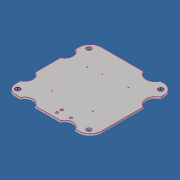
# Autodesk Inventor part: Eagle PCB rev 21
Saved by Autodesk Inventor 2016 (Build 200138000, 138)
## iProperties
Created: 2015-07-16
Part Number: Eagle PCB rev 21
Material: Generic
Document SubType Name: Modeling
Designer: Samuel Clay
Density: 1 g/cm^3
Appearance: Default
Author: Samuel Clay
Autodesk Inventor part; units mm, degrees
ref_plane "YZ Plane" through (0, 0, 0) normal (1, 0, 0) x (0, 1, 0)
ref_plane "XZ Plane" through (0, 0, 0) normal (0, 1, 0) x (-1, 0, 0)
ref_plane "XY Plane" through (0, 0, 0) normal (0, 0, 1) x (1, 0, 0)
sketch "Sketch1" plane through (0, 0, 0) normal (0, 0, 1) x (1, 0, 0)
  point P0 (0, 0)
sketch "0" plane through (0, 0, 0) normal (0, 1, 0) x (-1, 0, 0)
  line L0 (13.7795, -8.8674) -> (14.0221, -8.6401)
  line L1 (-19.1035, -9.4795) -> (-18.8376, -9.6291)
  line L2 (-20.445, -8.2504) -> (-20.2566, -8.4904)
  line L3 (3.0378, 26.1029) -> (3.2455, 25.8302)
  line L4 (3.2455, 25.8302) -> (3.4787, 25.5788)
  line L5 (-20.6394, 24.162) -> (-20.7961, 23.8688)
  line L6 (14.6382, 14.4375) -> (14.9109, 14.2297)
  line L7 (13.5247, 16.1335) -> (13.6387, 15.8102)
  line L8 (13.4425, 17.8296) -> (13.3929, 17.4904)
  line L9 (-21.0504, 23.2549) -> (-21.1469, 22.9368)
  line L10 (-19.8321, 25.2141) -> (-20.0593, 24.9715)
  line L11 (-19.5894, 25.4413) -> (-19.8321, 25.2141)
  line L12 (14.3869, 14.6706) -> (14.6382, 14.4375)
  line L13 (-16.5722, 26.6911) -> (-16.903, 26.6585)
  line L14 (-17.1381, 24.416) -> (-17.51, 24.7879)
  line L15 (-17.51, 24.7879) -> (-18.018, 24.924)
  line L16 (-18.8979, 23.4) -> (-18.526, 23.0281)
  line L17 (-18.018, 24.924) -> (-18.526, 24.7879)
  line L18 (-18.526, 24.7879) -> (-18.8979, 24.416)
  line L19 (-18.8979, 24.416) -> (-19.034, 23.908)
  line L20 (-19.034, 23.908) -> (-18.8979, 23.4)
  line L21 (-18.526, 23.0281) -> (-18.018, 22.892)
  line L22 (-18.018, 22.892) -> (-17.51, 23.0281)
  line L23 (14.3869, 19.6254) -> (14.1592, 19.369)
  line L24 (-19.0623, 25.8458) -> (-19.3325, 25.6522)
  line L25 (13.5247, 18.1624) -> (13.4425, 17.8296)
  line L26 (-20.2702, 24.7145) -> (-20.4638, 24.4443)
  line L27 (13.4425, 16.4663) -> (13.5247, 16.1335)
  line L28 (13.7834, 15.4994) -> (13.9574, 15.2041)
  line L29 (-19.3591, -9.3127) -> (-19.1035, -9.4795)
  line L30 (15.4666, -5.7111) -> (15.4992, -5.3803)
  line L31 (-4.9959, 24.162) -> (-4.81, 23.976)
  line L32 (-4.556, 24.924) -> (-4.81, 24.8559)
  line L33 (-4.81, 24.8559) -> (-4.9959, 24.67)
  line L34 (-4.9959, 24.67) -> (-5.064, 24.416)
  line L35 (-5.064, 24.416) -> (-4.9959, 24.162)
  line L36 (-4.81, 23.976) -> (-4.556, 23.908)
  line L37 (-4.556, 23.908) -> (-4.302, 23.976)
  line L38 (-4.302, 23.976) -> (-4.116, 24.162)
  line L39 (-4.116, 24.162) -> (-4.048, 24.416)
  line L40 (-10.487, -0.73) -> (-10.5091, -0.6475)
  line L41 (-10.5091, -0.8125) -> (-10.487, -0.73)
  line L42 (-10.5695, -0.8729) -> (-10.5091, -0.8125)
  line L43 (-10.652, -0.895) -> (-10.5695, -0.8729)
  line L44 (-10.7345, -0.8729) -> (-10.652, -0.895)
  line L45 (-10.7949, -0.8125) -> (-10.7345, -0.8729)
  line L46 (-10.817, -0.73) -> (-10.7949, -0.8125)
  line L47 (-10.7949, -0.6475) -> (-10.817, -0.73)
  line L48 (-10.7345, -0.5871) -> (-10.7949, -0.6475)
  line L49 (-10.652, -0.565) -> (-10.7345, -0.5871)
  line L50 (-10.5695, -0.5871) -> (-10.652, -0.565)
  line L51 (-10.5091, -0.6475) -> (-10.5695, -0.5871)
  line L52 (-18.2793, -9.8747) -> (-17.9893, -9.9696)
  line L53 (4.842, 17.469) -> (4.7595, 17.4469)
  line L54 (4.7595, 17.4469) -> (4.6991, 17.3865)
  line L55 (4.6991, 17.3865) -> (4.677, 17.304)
  line L56 (4.677, 17.304) -> (4.6991, 17.2215)
  line L57 (4.7595, 17.1611) -> (4.842, 17.139)
  line L58 (4.842, 17.139) -> (4.9245, 17.1611)
  line L59 (4.9245, 17.1611) -> (4.9849, 17.2215)
  line L60 (4.9849, 17.2215) -> (5.007, 17.304)
  line L61 (-21.32, -4.136) -> (-21.32, -6.0009)
  line L62 (-9.89, 22.96) -> (-9.636, 22.892)
  line L63 (-9.636, 22.892) -> (-9.382, 22.96)
  line L64 (-9.382, 22.96) -> (-9.196, 23.146)
  line L65 (-9.196, 23.146) -> (-9.128, 23.4)
  line L66 (-9.128, 23.4) -> (-9.196, 23.654)
  line L67 (-10.0759, 23.146) -> (-9.89, 22.96)
  line L68 (-10.144, 23.4) -> (-10.0759, 23.146)
  line L69 (-10.0759, 23.654) -> (-10.144, 23.4)
  line L70 (-9.89, 23.8399) -> (-10.0759, 23.654)
  line L71 (-9.636, 23.908) -> (-9.89, 23.8399)
  line L72 (-9.382, 23.8399) -> (-9.636, 23.908)
  line L73 (-9.196, 23.654) -> (-9.382, 23.8399)
  line L74 (4.3075, 24.9753) -> (4.6183, 24.8306)
  line L75 (14.4603, -8.1405) -> (14.6539, -7.8703)
  line L76 (14.6539, -7.8703) -> (14.8294, -7.588)
  line L77 (-17.9893, -9.9696) -> (-17.6937, -10.0453)
  line L78 (-8.8595, 25.8302) -> (-8.6517, 26.1029)
  line L79 (-8.6517, 26.1029) -> (-8.4713, 26.3944)
  line L80 (12.0629, -9.8584) -> (12.3741, -9.7413)
  line L81 (-18.5625, -9.761) -> (-18.2793, -9.8747)
  line L82 (-19.542, -7.08) -> (-19.4059, -7.588)
  line L83 (15.51, -5.048) -> (15.51, -3.628)
  line L84 (14.8294, -7.588) -> (14.9861, -7.2949)
  line L85 (14.9861, -7.2949) -> (15.1233, -6.9921)
  line L86 (15.1233, -6.9921) -> (15.2404, -6.6809)
  line L87 (14.0221, -8.6401) -> (14.2494, -8.3975)
  line L88 (-19.4059, -7.588) -> (-19.034, -7.9599)
  line L89 (-18.526, -6.064) -> (-19.034, -6.2002)
  line L90 (-19.034, -6.2002) -> (-19.4059, -6.572)
  line L91 (-17.0909, -10.1381) -> (-16.7862, -10.1547)
  line L92 (-4.302, 24.8559) -> (-4.556, 24.924)
  line L93 (-8.4713, 26.3944) -> (-8.32, 26.702)
  line L94 (-17.51, -7.08) -> (-17.6461, -6.572)
  line L95 (-14.4882, 26.1029) -> (-14.2805, 25.8302)
  line L96 (-12.5844, 24.7167) -> (-12.2516, 24.6345)
  line L97 (-14.6686, 26.3944) -> (-14.4882, 26.1029)
  line L98 (-19.4059, -6.572) -> (-19.542, -7.08)
  line L99 (7.2938, 24.8306) -> (7.6046, 24.9753)
  line L100 (4.9245, 17.4469) -> (4.842, 17.469)
  line L101 (4.6991, 17.2215) -> (4.7595, 17.1611)
  line L102 (14.2494, -8.3975) -> (14.4603, -8.1405)
  line L103 (-13.5139, 25.1494) -> (-13.2185, 24.9753)
  line L104 (-13.2185, 24.9753) -> (-12.9077, 24.8306)
  line L105 (2.706, 26.702) -> (2.8574, 26.3944)
  line L106 (15.3369, -6.3628) -> (15.4124, -6.0391)
  line L107 (15.4124, -6.0391) -> (15.4666, -5.7111)
  line L108 (-16.7862, -10.1547) -> (-16.4811, -10.1513)
  line L109 (-9.9214, 24.9753) -> (-9.6261, 25.1494)
  line L110 (-13.791, 25.3512) -> (-13.5139, 25.1494)
  line L111 (-14.82, 26.702) -> (-14.6686, 26.3944)
  line L112 (-17.6937, -10.0453) -> (-17.3938, -10.1016)
  line L113 (6.6377, 24.6345) -> (6.9705, 24.7167)
  line L114 (6.9705, 24.7167) -> (7.2938, 24.8306)
  line L115 (-20.0529, -8.7176) -> (-19.8348, -8.931)
  line L116 (-11.8395, 16.1769) -> (-11.922, 16.199)
  line L117 (-12.0649, 15.9515) -> (-12.0045, 15.8911)
  line L118 (-11.922, 16.199) -> (-12.0045, 16.1769)
  line L119 (-11.9124, 24.5849) -> (-11.57, 24.5683)
  line L120 (-11.57, 24.5683) -> (-11.2276, 24.5849)
  line L121 (4.6183, 24.8306) -> (4.9416, 24.7167)
  line L122 (7.6046, 24.9753) -> (7.8999, 25.1494)
  line L123 (4.9416, 24.7167) -> (5.2744, 24.6345)
  line L124 (-20.6173, -7.9986) -> (-20.445, -8.2504)
  line L125 (-21.32, 21.622) -> (-21.32, 3.38)
  line L126 (-12.0045, 16.1769) -> (-12.0649, 16.1165)
  line L127 (-12.0649, 16.1165) -> (-12.087, 16.034)
  line L128 (-11.757, 16.034) -> (-11.7791, 16.1165)
  line L129 (-11.7791, 15.9515) -> (-11.757, 16.034)
  line L130 (-11.8395, 15.8911) -> (-11.7791, 15.9515)
  line L131 (-11.922, 15.869) -> (-11.8395, 15.8911)
  line L132 (-12.0045, 15.8911) -> (-11.922, 15.869)
  line L133 (-12.087, 16.034) -> (-12.0649, 15.9515)
  line L134 (-11.7791, 16.1165) -> (-11.8395, 16.1769)
  line L135 (4.9849, 17.3865) -> (4.9245, 17.4469)
  line L136 (5.007, 17.304) -> (4.9849, 17.3865)
  line L137 (-16.1769, -10.128) -> (-15.328, -10.128)
  line L138 (3.735, 25.3512) -> (4.0121, 25.1494)
  line L139 (4.0121, 25.1494) -> (4.3075, 24.9753)
  line L140 (5.6136, 24.5849) -> (5.956, 24.5683)
  line L141 (5.956, 24.5683) -> (6.2984, 24.5849)
  line L142 (2.8574, 26.3944) -> (3.0378, 26.1029)
  line L143 (-17.6461, -7.588) -> (-17.51, -7.08)
  line L144 (-18.018, -7.9599) -> (-17.6461, -7.588)
  line L145 (-18.526, -8.096) -> (-18.018, -7.9599)
  line L146 (-19.034, -7.9599) -> (-18.526, -8.096)
  line L147 (-18.018, -6.2002) -> (-18.526, -6.064)
  line L148 (-17.6461, -6.572) -> (-18.018, -6.2002)
  line L149 (13.5225, -9.0783) -> (13.7795, -8.8674)
  line L150 (-20.7727, -7.736) -> (-20.6173, -7.9986)
  line L151 (-4.048, 22.384) -> (-4.116, 22.638)
  line L152 (6.277, 0.54) -> (6.2549, 0.6225)
  line L153 (6.2549, 0.4575) -> (6.277, 0.54)
  line L154 (6.1945, 0.3971) -> (6.2549, 0.4575)
  line L155 (6.112, 0.375) -> (6.1945, 0.3971)
  line L156 (6.0295, 0.3971) -> (6.112, 0.375)
  line L157 (5.9691, 0.4575) -> (6.0295, 0.3971)
  line L158 (5.947, 0.54) -> (5.9691, 0.4575)
  line L159 (5.9691, 0.6225) -> (5.947, 0.54)
  line L160 (6.0295, 0.6829) -> (5.9691, 0.6225)
  line L161 (6.112, 0.705) -> (6.0295, 0.6829)
  line L162 (6.1945, 0.6829) -> (6.112, 0.705)
  line L163 (6.2549, 0.6225) -> (6.1945, 0.6829)
  line L164 (8.4334, 25.5788) -> (8.6665, 25.8302)
  line L165 (8.6665, 25.8302) -> (8.8743, 26.1029)
  line L166 (-4.116, 22.638) -> (-4.302, 22.8239)
  line L167 (-20.2566, -8.4904) -> (-20.0529, -8.7176)
  line L168 (-4.302, 22.8239) -> (-4.556, 22.892)
  line L169 (-4.9959, 22.13) -> (-4.81, 21.944)
  line L170 (-4.556, 22.892) -> (-4.81, 22.8239)
  line L171 (-4.81, 22.8239) -> (-4.9959, 22.638)
  line L172 (-4.9959, 22.638) -> (-5.064, 22.384)
  line L173 (-5.064, 22.384) -> (-4.9959, 22.13)
  line L174 (-4.81, 21.944) -> (-4.556, 21.876)
  line L175 (-4.556, 21.876) -> (-4.302, 21.944)
  line L176 (-4.302, 21.944) -> (-4.116, 22.13)
  line L177 (-4.116, 22.13) -> (-4.048, 22.384)
  line L178 (13.2435, 26.2829) -> (13.0013, 26.3926)
  line L179 (13.0013, 26.3926) -> (12.7524, 26.4863)
  line L180 (-20.0212, -3.2426) -> (-19.758, -2.9462)
  line L181 (-19.758, -2.9462) -> (-19.5247, -2.6258)
  line L182 (-19.5247, -2.6258) -> (-19.3234, -2.2843)
  line L183 (-15.1529, -9.7724) -> (-15.328, -10.128)
  line L184 (15.2024, -3.4767) -> (15.51, -3.628)
  line L185 (-14.9443, -9.4353) -> (-15.1529, -9.7724)
  line L186 (13.6387, 0.9597) -> (13.5247, 0.6364)
  line L187 (-14.7041, -9.1199) -> (-14.9443, -9.4353)
  line L188 (14.9109, -3.2963) -> (15.2024, -3.4767)
  line L189 (-14.4346, -8.8293) -> (-14.7041, -9.1199)
  line L190 (13.7834, 1.2705) -> (13.6387, 0.9597)
  line L191 (-14.1382, -8.5661) -> (-14.4346, -8.8293)
  line L192 (-13.8177, -8.3328) -> (-14.1382, -8.5661)
  line L193 (14.6382, -3.0885) -> (14.9109, -3.2963)
  line L194 (-13.4762, -8.1315) -> (-13.8177, -8.3328)
  line L195 (14.3869, -2.8554) -> (14.6382, -3.0885)
  line L196 (-13.1168, -7.9642) -> (-13.4762, -8.1315)
  line L197 (-12.743, -7.8324) -> (-13.1168, -7.9642)
  line L198 (-12.3581, -7.7374) -> (-12.743, -7.8324)
  line L199 (-11.9659, -7.68) -> (-12.3581, -7.7374)
  line L200 (13.9574, 1.5659) -> (13.7834, 1.2705)
  line L201 (14.1592, -2.5991) -> (14.3869, -2.8554)
  line L202 (-11.57, -7.6608) -> (-11.9659, -7.68)
  line L203 (13.9574, -2.3219) -> (14.1592, -2.5991)
  line L204 (-11.174, -7.68) -> (-11.57, -7.6608)
  line L205 (14.1592, 1.843) -> (13.9574, 1.5659)
  line L206 (13.7834, -2.0266) -> (13.9574, -2.3219)
  line L207 (-10.7818, -7.7374) -> (-11.174, -7.68)
  line L208 (14.3869, 2.0993) -> (14.1592, 1.843)
  line L209 (-10.397, -7.8324) -> (-10.7818, -7.7374)
  line L210 (-10.0231, -7.9642) -> (-10.397, -7.8324)
  line L211 (-9.6637, -8.1315) -> (-10.0231, -7.9642)
  line L212 (-9.3222, -8.3328) -> (-9.6637, -8.1315)
  line L213 (14.6382, 2.3325) -> (14.3869, 2.0993)
  line L214 (13.6387, -1.7158) -> (13.7834, -2.0266)
  line L215 (-9.0018, -8.5661) -> (-9.3222, -8.3328)
  line L216 (-8.7054, -8.8293) -> (-9.0018, -8.5661)
  line L217 (13.5247, -1.3925) -> (13.6387, -1.7158)
  line L218 (14.9109, 2.5402) -> (14.6382, 2.3325)
  line L219 (-8.4358, -9.1199) -> (-8.7054, -8.8293)
  line L220 (13.4425, -1.0597) -> (13.5247, -1.3925)
  line L221 (-8.1956, -9.4353) -> (-8.4358, -9.1199)
  line L222 (15.2024, 2.7206) -> (14.9109, 2.5402)
  line L223 (-7.987, -9.7724) -> (-8.1956, -9.4353)
  line L224 (13.3929, -0.7205) -> (13.4425, -1.0597)
  line L225 (-7.812, -10.128) -> (-7.987, -9.7724)
  line L226 (-20.9643, 3.2049) -> (-21.32, 3.38)
  line L227 (13.3763, -0.378) -> (13.3929, -0.7205)
  line L228 (-20.6272, 2.9963) -> (-20.9643, 3.2049)
  line L229 (-20.3119, 2.7561) -> (-20.6272, 2.9963)
  line L230 (-20.0212, 2.4866) -> (-20.3119, 2.7561)
  line L231 (13.3929, -0.0356) -> (13.3763, -0.378)
  line L232 (-19.758, 2.1902) -> (-20.0212, 2.4866)
  line L233 (15.51, 2.872) -> (15.2024, 2.7206)
  line L234 (13.4425, 0.3036) -> (13.3929, -0.0356)
  line L235 (13.5247, 0.6364) -> (13.4425, 0.3036)
  line L236 (-19.5247, 1.8697) -> (-19.758, 2.1902)
  line L237 (-19.3234, 1.5282) -> (-19.5247, 1.8697)
  line L238 (-20.9333, 23.566) -> (-21.0504, 23.2549)
  line L239 (13.9574, 15.2041) -> (14.1592, 14.9269)
  line L240 (-17.002, 23.908) -> (-17.1381, 24.416)
  line L241 (-21.3091, 21.9542) -> (-21.32, 21.622)
  line L242 (-17.1381, 23.4) -> (-17.002, 23.908)
  line L243 (-17.51, 23.0281) -> (-17.1381, 23.4)
  line L244 (-20.4638, 24.4443) -> (-20.6394, 24.162)
  line L245 (14.6382, 19.8585) -> (14.3869, 19.6254)
  line L246 (15.51, 20.398) -> (15.2024, 20.2466)
  line L247 (-17.8729, 26.4324) -> (-18.184, 26.3153)
  line L248 (13.3929, 16.8056) -> (13.4425, 16.4663)
  line L249 (-20.7961, 23.8688) -> (-20.9333, 23.566)
  line L250 (-18.4868, 26.1781) -> (-18.78, 26.0214)
  line L251 (-18.78, 26.0214) -> (-19.0623, 25.8458)
  line L252 (-21.1469, 22.9368) -> (-21.2224, 22.613)
  line L253 (13.732, -6.826) -> (13.5959, -6.318)
  line L254 (13.3763, 17.148) -> (13.3929, 16.8056)
  line L255 (13.3929, 17.4904) -> (13.3763, 17.148)
  line L256 (-18.184, 26.3153) -> (-18.4868, 26.1781)
  line L257 (-19.3325, 25.6522) -> (-19.5894, 25.4413)
  line L258 (14.1592, 19.369) -> (13.9574, 19.0919)
  line L259 (13.6387, 15.8102) -> (13.7834, 15.4994)
  line L260 (-21.2765, 22.285) -> (-21.3091, 21.9542)
  line L261 (-21.2224, 22.613) -> (-21.2765, 22.285)
  line L262 (-17.5548, 26.5289) -> (-17.8729, 26.4324)
  line L263 (-20.0593, 24.9715) -> (-20.2702, 24.7145)
  line L264 (-17.231, 26.6044) -> (-17.5548, 26.5289)
  line L265 (15.2024, 20.2466) -> (14.9109, 20.0662)
  line L266 (14.9109, 20.0662) -> (14.6382, 19.8585)
  line L267 (-16.24, 26.702) -> (-16.5722, 26.6911)
  line L268 (-16.903, 26.6585) -> (-17.231, 26.6044)
  line L269 (14.9109, 14.2297) -> (15.2024, 14.0493)
  line L270 (15.2024, 14.0493) -> (15.51, 13.898)
  line L271 (13.5959, -6.318) -> (13.224, -5.9462)
  line L272 (13.224, -5.9462) -> (12.716, -5.81)
  line L273 (11.8362, -7.334) -> (12.208, -7.7059)
  line L274 (14.1592, 14.9269) -> (14.3869, 14.6706)
  line L275 (13.6387, 18.4857) -> (13.5247, 18.1624)
  line L276 (13.9574, 19.0919) -> (13.7834, 18.7965)
  line L277 (13.7834, 18.7965) -> (13.6387, 18.4857)
  line L278 (12.716, -5.81) -> (12.208, -5.9462)
  line L279 (12.208, -5.9462) -> (11.8362, -6.318)
  line L280 (11.8362, -6.318) -> (11.7, -6.826)
  line L281 (11.7, -6.826) -> (11.8362, -7.334)
  line L282 (12.208, -7.7059) -> (12.716, -7.842)
  line L283 (12.716, -7.842) -> (13.224, -7.7059)
  line L284 (13.224, -7.7059) -> (13.5959, -7.334)
  line L285 (13.5959, -7.334) -> (13.732, -6.826)
  line L286 (13.986, 24.162) -> (13.8499, 24.67)
  line L287 (13.8499, 24.67) -> (13.478, 25.0419)
  line L288 (13.478, 25.0419) -> (12.97, 25.178)
  line L289 (12.0902, 23.654) -> (12.462, 23.2821)
  line L290 (12.97, 25.178) -> (12.462, 25.0419)
  line L291 (12.462, 25.0419) -> (12.0902, 24.67)
  line L292 (12.0902, 24.67) -> (11.954, 24.162)
  line L293 (11.954, 24.162) -> (12.0902, 23.654)
  line L294 (12.462, 23.2821) -> (12.97, 23.146)
  line L295 (-14.82, 26.702) -> (-16.24, 26.702)
  line L296 (12.97, 23.146) -> (13.478, 23.2821)
  line L297 (13.478, 23.2821) -> (13.8499, 23.654)
  line L298 (13.8499, 23.654) -> (13.986, 24.162)
  line L299 (-14.2805, 25.8302) -> (-14.0473, 25.5788)
  line L300 (-14.0473, 25.5788) -> (-13.791, 25.3512)
  line L301 (-12.9077, 24.8306) -> (-12.5844, 24.7167)
  line L302 (-12.2516, 24.6345) -> (-11.9124, 24.5849)
  line L303 (-11.2276, 24.5849) -> (-10.8883, 24.6345)
  line L304 (-10.8883, 24.6345) -> (-10.5555, 24.7167)
  line L305 (-10.5555, 24.7167) -> (-10.2322, 24.8306)
  line L306 (-10.2322, 24.8306) -> (-9.9214, 24.9753)
  line L307 (-9.6261, 25.1494) -> (-9.3489, 25.3512)
  line L308 (-9.3489, 25.3512) -> (-9.0926, 25.5788)
  line L309 (-9.0926, 25.5788) -> (-8.8595, 25.8302)
  line L310 (2.706, 26.702) -> (-8.32, 26.702)
  line L311 (3.4787, 25.5788) -> (3.735, 25.3512)
  line L312 (5.2744, 24.6345) -> (5.6136, 24.5849)
  line L313 (6.2984, 24.5849) -> (6.6377, 24.6345)
  line L314 (7.8999, 25.1494) -> (8.1771, 25.3512)
  line L315 (8.1771, 25.3512) -> (8.4334, 25.5788)
  line L316 (8.8743, 26.1029) -> (9.0547, 26.3944)
  line L317 (9.0547, 26.3944) -> (9.206, 26.702)
  line L318 (11.446, 26.702) -> (9.206, 26.702)
  line L319 (11.7118, 26.6933) -> (11.446, 26.702)
  line L320 (11.9765, 26.6672) -> (11.7118, 26.6933)
  line L321 (12.2389, 26.6239) -> (11.9765, 26.6672)
  line L322 (12.4979, 26.5635) -> (12.2389, 26.6239)
  line L323 (12.7524, 26.4863) -> (12.4979, 26.5635)
  line L324 (13.478, 26.1575) -> (13.2435, 26.2829)
  line L325 (13.7039, 26.0171) -> (13.478, 26.1575)
  line L326 (13.92, 25.8622) -> (13.7039, 26.0171)
  line L327 (14.1256, 25.6935) -> (13.92, 25.8622)
  line L328 (14.3197, 25.5117) -> (14.1256, 25.6935)
  line L329 (14.5015, 25.3176) -> (14.3197, 25.5117)
  line L330 (14.6702, 25.112) -> (14.5015, 25.3176)
  line L331 (14.8251, 24.8958) -> (14.6702, 25.112)
  line L332 (14.9656, 24.67) -> (14.8251, 24.8958)
  line L333 (15.0909, 24.4354) -> (14.9656, 24.67)
  line L334 (15.2007, 24.1932) -> (15.0909, 24.4354)
  line L335 (15.2944, 23.9443) -> (15.2007, 24.1932)
  line L336 (15.3716, 23.6898) -> (15.2944, 23.9443)
  line L337 (15.4319, 23.4308) -> (15.3716, 23.6898)
  line L338 (15.4753, 23.1684) -> (15.4319, 23.4308)
  line L339 (15.5013, 22.9038) -> (15.4753, 23.1684)
  line L340 (15.51, 22.638) -> (15.5013, 22.9038)
  line L341 (15.51, 20.398) -> (15.51, 22.638)
  line L342 (15.51, 2.872) -> (15.51, 13.898)
  line L343 (15.4992, -5.3803) -> (15.51, -5.048)
  line L344 (15.2404, -6.6809) -> (15.3369, -6.3628)
  line L345 (13.2523, -9.2719) -> (13.5225, -9.0783)
  line L346 (12.97, -9.4474) -> (13.2523, -9.2719)
  line L347 (12.6769, -9.6041) -> (12.97, -9.4474)
  line L348 (12.3741, -9.7413) -> (12.6769, -9.6041)
  line L349 (11.7448, -9.9549) -> (12.0629, -9.8584)
  line L350 (11.4211, -10.0304) -> (11.7448, -9.9549)
  line L351 (11.0931, -10.0846) -> (11.4211, -10.0304)
  line L352 (10.7623, -10.1172) -> (11.0931, -10.0846)
  line L353 (10.43, -10.128) -> (10.7623, -10.1172)
  line L354 (-7.812, -10.128) -> (10.43, -10.128)
  line L355 (-16.4811, -10.1513) -> (-16.1769, -10.128)
  line L356 (-17.3938, -10.1016) -> (-17.0909, -10.1381)
  line L357 (-18.8376, -9.6291) -> (-18.5625, -9.761)
  line L358 (-19.6032, -9.1297) -> (-19.3591, -9.3127)
  line L359 (-19.8348, -8.931) -> (-19.6032, -9.1297)
  line L360 (-20.9107, -7.4639) -> (-20.7727, -7.736)
  line L361 (-21.0306, -7.1833) -> (-20.9107, -7.4639)
  line L362 (-21.1318, -6.8954) -> (-21.0306, -7.1833)
  line L363 (-21.214, -6.6016) -> (-21.1318, -6.8954)
  line L364 (-21.2768, -6.303) -> (-21.214, -6.6016)
  line L365 (-21.32, -6.0009) -> (-21.2768, -6.303)
  line L366 (-21.32, -4.136) -> (-20.9643, -3.961)
  line L367 (-20.9643, -3.961) -> (-20.6272, -3.7524)
  line L368 (-20.6272, -3.7524) -> (-20.3119, -3.5122)
  line L369 (-20.3119, -3.5122) -> (-20.0212, -3.2426)
  line L370 (-19.3234, -2.2843) -> (-19.1561, -1.9249)
  line L371 (-19.1561, -1.9249) -> (-19.0243, -1.551)
  line L372 (-19.0243, -1.551) -> (-18.9293, -1.1662)
  line L373 (-18.9293, -1.1662) -> (-18.872, -0.774)
  line L374 (-18.872, -0.774) -> (-18.8528, -0.378)
  line L375 (-18.8528, -0.378) -> (-18.872, 0.0179)
  line L376 (-18.872, 0.0179) -> (-18.9293, 0.4101)
  line L377 (-18.9293, 0.4101) -> (-19.0243, 0.795)
  line L378 (-19.0243, 0.795) -> (-19.1561, 1.1688)
  line L379 (-19.1561, 1.1688) -> (-19.3234, 1.5282)
  line L380 (-4.048, 24.416) -> (-4.116, 24.67)
  line L381 (-4.116, 24.67) -> (-4.302, 24.8559)
  dimension "d0" = 36.83
  constraints: 764 end point, 165 perpendicular, 137 parallel, 4 collinear
  measures "d0" distance between parallel lines of L342 L125
extrude "Extrusion1" add sketch "0" along normal blind 0.7112
sketch "Sketch3" plane through (0, 0.7112, 0) normal (0, 1, 0) x (1, 0, 0)
  line L0 (-13.986, -24.162) -> (-13.8499, -23.654) projected
  line L1 (-13.8499, -23.654) -> (-13.478, -23.2821) projected
  line L2 (-13.478, -23.2821) -> (-12.97, -23.146) projected
  line L3 (-12.97, -23.146) -> (-12.462, -23.2821) projected
  line L4 (-12.462, -23.2821) -> (-12.0902, -23.654) projected
  line L5 (-12.0902, -23.654) -> (-11.954, -24.162) projected
  line L6 (-11.954, -24.162) -> (-12.0902, -24.67) projected
  line L7 (-12.0902, -24.67) -> (-12.462, -25.0419) projected
  line L8 (-12.462, -25.0419) -> (-12.97, -25.178) projected
  line L9 (-12.97, -25.178) -> (-13.478, -25.0419) projected
  line L10 (-13.478, -25.0419) -> (-13.8499, -24.67) projected
  line L11 (-13.8499, -24.67) -> (-13.986, -24.162) projected
  line L12 (-13.732, 6.826) -> (-13.5959, 7.334) projected
  line L13 (-13.5959, 7.334) -> (-13.224, 7.7059) projected
  line L14 (-13.224, 7.7059) -> (-12.716, 7.842) projected
  line L15 (-12.716, 7.842) -> (-12.208, 7.7059) projected
  line L16 (-12.208, 7.7059) -> (-11.8362, 7.334) projected
  line L17 (-11.8362, 7.334) -> (-11.7, 6.826) projected
  line L18 (-11.7, 6.826) -> (-11.8362, 6.318) projected
  line L19 (-11.8362, 6.318) -> (-12.208, 5.9462) projected
  line L20 (-12.208, 5.9462) -> (-12.716, 5.81) projected
  line L21 (-12.716, 5.81) -> (-13.224, 5.9462) projected
  line L22 (-13.224, 5.9462) -> (-13.5959, 6.318) projected
  line L23 (-13.5959, 6.318) -> (-13.732, 6.826) projected
  line L24 (19.542, 7.08) -> (19.4059, 6.572) projected
  line L25 (19.4059, 6.572) -> (19.034, 6.2002) projected
  line L26 (19.034, 6.2002) -> (18.526, 6.064) projected
  line L27 (18.526, 6.064) -> (18.018, 6.2002) projected
  line L28 (18.018, 6.2002) -> (17.6461, 6.572) projected
  line L29 (17.6461, 6.572) -> (17.51, 7.08) projected
  line L30 (17.51, 7.08) -> (17.6461, 7.588) projected
  line L31 (17.6461, 7.588) -> (18.018, 7.9599) projected
  line L32 (18.018, 7.9599) -> (18.526, 8.096) projected
  line L33 (18.526, 8.096) -> (19.034, 7.9599) projected
  line L34 (19.034, 7.9599) -> (19.4059, 7.588) projected
  line L35 (19.4059, 7.588) -> (19.542, 7.08) projected
  line L36 (17.1381, -24.416) -> (17.002, -23.908) projected
  line L37 (17.002, -23.908) -> (17.1381, -23.4) projected
  line L38 (17.1381, -23.4) -> (17.51, -23.0281) projected
  line L39 (17.51, -23.0281) -> (18.018, -22.892) projected
  line L40 (18.018, -22.892) -> (18.526, -23.0281) projected
  line L41 (18.526, -23.0281) -> (18.8979, -23.4) projected
  line L42 (18.8979, -23.4) -> (19.034, -23.908) projected
  line L43 (19.034, -23.908) -> (18.8979, -24.416) projected
  line L44 (18.8979, -24.416) -> (18.526, -24.7879) projected
  line L45 (18.526, -24.7879) -> (18.018, -24.924) projected
  line L46 (18.018, -24.924) -> (17.51, -24.7879) projected
  line L47 (17.51, -24.7879) -> (17.1381, -24.416) projected
  line L48 (4.048, -22.384) -> (4.116, -22.13) projected
  line L49 (4.116, -22.13) -> (4.302, -21.944) projected
  line L50 (4.302, -21.944) -> (4.556, -21.876) projected
  line L51 (4.556, -21.876) -> (4.81, -21.944) projected
  line L52 (4.81, -21.944) -> (4.9959, -22.13) projected
  line L53 (4.9959, -22.13) -> (5.064, -22.384) projected
  line L54 (5.064, -22.384) -> (4.9959, -22.638) projected
  line L55 (4.9959, -22.638) -> (4.81, -22.8239) projected
  line L56 (4.81, -22.8239) -> (4.556, -22.892) projected
  line L57 (4.556, -22.892) -> (4.302, -22.8239) projected
  line L58 (4.302, -22.8239) -> (4.116, -22.638) projected
  line L59 (4.116, -22.638) -> (4.048, -22.384) projected
  line L60 (9.89, -22.96) -> (10.0759, -23.146) projected
  line L61 (10.0759, -23.146) -> (10.144, -23.4) projected
  line L62 (10.144, -23.4) -> (10.0759, -23.654) projected
  line L63 (10.0759, -23.654) -> (9.89, -23.8399) projected
  line L64 (9.89, -23.8399) -> (9.636, -23.908) projected
  line L65 (9.636, -23.908) -> (9.382, -23.8399) projected
  line L66 (9.382, -23.8399) -> (9.196, -23.654) projected
  line L67 (9.196, -23.654) -> (9.128, -23.4) projected
  line L68 (9.128, -23.4) -> (9.196, -23.146) projected
  line L69 (9.196, -23.146) -> (9.382, -22.96) projected
  line L70 (9.382, -22.96) -> (9.636, -22.892) projected
  line L71 (9.636, -22.892) -> (9.89, -22.96) projected
  line L72 (4.9959, -24.162) -> (5.064, -24.416) projected
  line L73 (5.064, -24.416) -> (4.9959, -24.67) projected
  line L74 (4.9959, -24.67) -> (4.81, -24.8559) projected
  line L75 (4.81, -24.8559) -> (4.556, -24.924) projected
  line L76 (4.556, -24.924) -> (4.302, -24.8559) projected
  line L77 (4.302, -24.8559) -> (4.116, -24.67) projected
  line L78 (4.116, -24.67) -> (4.048, -24.416) projected
  line L79 (4.048, -24.416) -> (4.116, -24.162) projected
  line L80 (4.116, -24.162) -> (4.302, -23.976) projected
  line L81 (4.302, -23.976) -> (4.556, -23.908) projected
  line L82 (4.556, -23.908) -> (4.81, -23.976) projected
  line L83 (4.81, -23.976) -> (4.9959, -24.162) projected
  line L84 (-6.277, -0.54) -> (-6.2549, -0.4575) projected
  line L85 (-6.2549, -0.4575) -> (-6.1945, -0.3971) projected
  line L86 (-6.1945, -0.3971) -> (-6.112, -0.375) projected
  line L87 (-6.112, -0.375) -> (-6.0295, -0.3971) projected
  line L88 (-6.0295, -0.3971) -> (-5.9691, -0.4575) projected
  line L89 (-5.9691, -0.4575) -> (-5.947, -0.54) projected
  line L90 (-5.947, -0.54) -> (-5.9691, -0.6225) projected
  line L91 (-5.9691, -0.6225) -> (-6.0295, -0.6829) projected
  line L92 (-6.0295, -0.6829) -> (-6.112, -0.705) projected
  line L93 (-6.112, -0.705) -> (-6.1945, -0.6829) projected
  line L94 (-6.1945, -0.6829) -> (-6.2549, -0.6225) projected
  line L95 (-6.2549, -0.6225) -> (-6.277, -0.54) projected
  line L96 (11.8395, -16.1769) -> (11.7791, -16.1165) projected
  line L97 (11.7791, -16.1165) -> (11.757, -16.034) projected
  line L98 (11.757, -16.034) -> (11.7791, -15.9515) projected
  line L99 (11.7791, -15.9515) -> (11.8395, -15.8911) projected
  line L100 (11.8395, -15.8911) -> (11.922, -15.869) projected
  line L101 (11.922, -15.869) -> (12.0045, -15.8911) projected
  line L102 (12.0045, -15.8911) -> (12.0649, -15.9515) projected
  line L103 (12.0649, -15.9515) -> (12.087, -16.034) projected
  line L104 (12.087, -16.034) -> (12.0649, -16.1165) projected
  line L105 (12.0649, -16.1165) -> (12.0045, -16.1769) projected
  line L106 (12.0045, -16.1769) -> (11.922, -16.199) projected
  line L107 (11.922, -16.199) -> (11.8395, -16.1769) projected
  line L108 (-4.842, -17.469) -> (-4.9245, -17.4469) projected
  line L109 (-4.9245, -17.4469) -> (-4.9849, -17.3865) projected
  line L110 (-4.9849, -17.3865) -> (-5.007, -17.304) projected
  line L111 (-5.007, -17.304) -> (-4.9849, -17.2215) projected
  line L112 (-4.9849, -17.2215) -> (-4.9245, -17.1611) projected
  line L113 (-4.9245, -17.1611) -> (-4.842, -17.139) projected
  line L114 (-4.842, -17.139) -> (-4.7595, -17.1611) projected
  line L115 (-4.7595, -17.1611) -> (-4.6991, -17.2215) projected
  line L116 (-4.6991, -17.2215) -> (-4.677, -17.304) projected
  line L117 (-4.677, -17.304) -> (-4.6991, -17.3865) projected
  line L118 (-4.6991, -17.3865) -> (-4.7595, -17.4469) projected
  line L119 (-4.7595, -17.4469) -> (-4.842, -17.469) projected
  line L120 (10.487, 0.73) -> (10.5091, 0.8125) projected
  line L121 (10.5091, 0.8125) -> (10.5695, 0.8729) projected
  line L122 (10.5695, 0.8729) -> (10.652, 0.895) projected
  line L123 (10.652, 0.895) -> (10.7345, 0.8729) projected
  line L124 (10.7345, 0.8729) -> (10.7949, 0.8125) projected
  line L125 (10.7949, 0.8125) -> (10.817, 0.73) projected
  line L126 (10.817, 0.73) -> (10.7949, 0.6475) projected
  line L127 (10.7949, 0.6475) -> (10.7345, 0.5871) projected
  line L128 (10.7345, 0.5871) -> (10.652, 0.565) projected
  line L129 (10.652, 0.565) -> (10.5695, 0.5871) projected
  line L130 (10.5695, 0.5871) -> (10.5091, 0.6475) projected
  line L131 (10.5091, 0.6475) -> (10.487, 0.73) projected
  line L132 (-13.7795, 8.8674) -> (-14.0221, 8.6401) projected
  line L133 (-14.0221, 8.6401) -> (-14.2494, 8.3975) projected
  line L134 (-14.2494, 8.3975) -> (-14.4603, 8.1405) projected
  line L135 (-14.4603, 8.1405) -> (-14.6539, 7.8703) projected
  line L136 (-14.6539, 7.8703) -> (-14.8294, 7.588) projected
  line L137 (-14.8294, 7.588) -> (-14.9861, 7.2949) projected
  line L138 (-14.9861, 7.2949) -> (-15.1233, 6.9921) projected
  line L139 (-15.1233, 6.9921) -> (-15.2404, 6.6809) projected
  line L140 (-15.2404, 6.6809) -> (-15.3369, 6.3628) projected
  line L141 (-15.3369, 6.3628) -> (-15.4124, 6.0391) projected
  line L142 (-15.4124, 6.0391) -> (-15.4666, 5.7111) projected
  line L143 (-15.4666, 5.7111) -> (-15.4992, 5.3803) projected
  line L144 (-15.4992, 5.3803) -> (-15.51, 5.048) projected
  line L145 (-15.51, 5.048) -> (-15.51, 3.628) projected
  line L146 (-15.51, 3.628) -> (-15.2024, 3.4767) projected
  line L147 (-15.2024, 3.4767) -> (-14.9109, 3.2963) projected
  line L148 (-14.9109, 3.2963) -> (-14.6382, 3.0885) projected
  line L149 (-14.6382, 3.0885) -> (-14.3869, 2.8554) projected
  line L150 (-14.3869, 2.8554) -> (-14.1592, 2.5991) projected
  line L151 (-14.1592, 2.5991) -> (-13.9574, 2.3219) projected
  line L152 (-13.9574, 2.3219) -> (-13.7834, 2.0266) projected
  line L153 (-13.7834, 2.0266) -> (-13.6387, 1.7158) projected
  line L154 (-13.6387, 1.7158) -> (-13.5247, 1.3925) projected
  line L155 (-13.5247, 1.3925) -> (-13.4425, 1.0597) projected
  line L156 (-13.4425, 1.0597) -> (-13.3929, 0.7205) projected
  line L157 (-13.3929, 0.7205) -> (-13.3763, 0.378) projected
  line L158 (-13.3763, 0.378) -> (-13.3929, 0.0356) projected
  line L159 (-13.3929, 0.0356) -> (-13.4425, -0.3036) projected
  line L160 (-13.4425, -0.3036) -> (-13.5247, -0.6364) projected
  line L161 (-13.5247, -0.6364) -> (-13.6387, -0.9597) projected
  line L162 (-13.6387, -0.9597) -> (-13.7834, -1.2705) projected
  line L163 (-13.7834, -1.2705) -> (-13.9574, -1.5659) projected
  line L164 (-13.9574, -1.5659) -> (-14.1592, -1.843) projected
  line L165 (-14.1592, -1.843) -> (-14.3869, -2.0993) projected
  line L166 (-14.3869, -2.0993) -> (-14.6382, -2.3325) projected
  line L167 (-14.6382, -2.3325) -> (-14.9109, -2.5402) projected
  line L168 (-14.9109, -2.5402) -> (-15.2024, -2.7206) projected
  line L169 (-15.2024, -2.7206) -> (-15.51, -2.872) projected
  line L170 (-15.51, -2.872) -> (-15.51, -13.898) projected
  line L171 (-15.51, -13.898) -> (-15.2024, -14.0493) projected
  line L172 (-15.2024, -14.0493) -> (-14.9109, -14.2297) projected
  line L173 (-14.9109, -14.2297) -> (-14.6382, -14.4375) projected
  line L174 (-14.6382, -14.4375) -> (-14.3869, -14.6706) projected
  line L175 (-14.3869, -14.6706) -> (-14.1592, -14.9269) projected
  line L176 (-14.1592, -14.9269) -> (-13.9574, -15.2041) projected
  line L177 (-13.9574, -15.2041) -> (-13.7834, -15.4994) projected
  line L178 (-13.7834, -15.4994) -> (-13.6387, -15.8102) projected
  line L179 (-13.6387, -15.8102) -> (-13.5247, -16.1335) projected
  line L180 (-13.5247, -16.1335) -> (-13.4425, -16.4663) projected
  line L181 (-13.4425, -16.4663) -> (-13.3929, -16.8056) projected
  line L182 (-13.3929, -16.8056) -> (-13.3763, -17.148) projected
  line L183 (-13.3763, -17.148) -> (-13.3929, -17.4904) projected
  line L184 (-13.3929, -17.4904) -> (-13.4425, -17.8296) projected
  line L185 (-13.4425, -17.8296) -> (-13.5247, -18.1624) projected
  line L186 (-13.5247, -18.1624) -> (-13.6387, -18.4857) projected
  line L187 (-13.6387, -18.4857) -> (-13.7834, -18.7965) projected
  line L188 (-13.7834, -18.7965) -> (-13.9574, -19.0919) projected
  line L189 (-13.9574, -19.0919) -> (-14.1592, -19.369) projected
  line L190 (-14.1592, -19.369) -> (-14.3869, -19.6254) projected
  line L191 (-14.3869, -19.6254) -> (-14.6382, -19.8585) projected
  line L192 (-14.6382, -19.8585) -> (-14.9109, -20.0662) projected
  line L193 (-14.9109, -20.0662) -> (-15.2024, -20.2466) projected
  line L194 (-15.2024, -20.2466) -> (-15.51, -20.398) projected
  line L195 (-15.51, -20.398) -> (-15.51, -22.638) projected
  line L196 (-15.51, -22.638) -> (-15.5013, -22.9038) projected
  line L197 (-15.5013, -22.9038) -> (-15.4753, -23.1684) projected
  line L198 (-15.4753, -23.1684) -> (-15.4319, -23.4308) projected
  line L199 (-15.4319, -23.4308) -> (-15.3716, -23.6898) projected
  line L200 (-15.3716, -23.6898) -> (-15.2944, -23.9443) projected
  line L201 (-15.2944, -23.9443) -> (-15.2007, -24.1932) projected
  line L202 (-15.2007, -24.1932) -> (-15.0909, -24.4354) projected
  line L203 (-15.0909, -24.4354) -> (-14.9656, -24.67) projected
  line L204 (-14.9656, -24.67) -> (-14.8251, -24.8958) projected
  line L205 (-14.8251, -24.8958) -> (-14.6702, -25.112) projected
  line L206 (-14.6702, -25.112) -> (-14.5015, -25.3176) projected
  line L207 (-14.5015, -25.3176) -> (-14.3197, -25.5117) projected
  line L208 (-14.3197, -25.5117) -> (-14.1256, -25.6935) projected
  line L209 (-14.1256, -25.6935) -> (-13.92, -25.8622) projected
  line L210 (-13.92, -25.8622) -> (-13.7039, -26.0171) projected
  line L211 (-13.7039, -26.0171) -> (-13.478, -26.1575) projected
  line L212 (-13.478, -26.1575) -> (-13.2435, -26.2829) projected
  line L213 (-13.2435, -26.2829) -> (-13.0013, -26.3926) projected
  line L214 (-13.0013, -26.3926) -> (-12.7524, -26.4863) projected
  line L215 (-12.7524, -26.4863) -> (-12.4979, -26.5635) projected
  line L216 (-12.4979, -26.5635) -> (-12.2389, -26.6239) projected
  line L217 (-12.2389, -26.6239) -> (-11.9765, -26.6672) projected
  line L218 (-11.9765, -26.6672) -> (-11.7118, -26.6933) projected
  line L219 (-11.7118, -26.6933) -> (-11.446, -26.702) projected
  line L220 (-11.446, -26.702) -> (-9.206, -26.702) projected
  line L221 (-9.206, -26.702) -> (-9.0547, -26.3944) projected
  line L222 (-9.0547, -26.3944) -> (-8.8743, -26.1029) projected
  line L223 (-8.8743, -26.1029) -> (-8.6665, -25.8302) projected
  line L224 (-8.6665, -25.8302) -> (-8.4334, -25.5788) projected
  line L225 (-8.4334, -25.5788) -> (-8.1771, -25.3512) projected
  line L226 (-8.1771, -25.3512) -> (-7.8999, -25.1494) projected
  line L227 (-7.8999, -25.1494) -> (-7.6046, -24.9753) projected
  line L228 (-7.6046, -24.9753) -> (-7.2938, -24.8306) projected
  line L229 (-7.2938, -24.8306) -> (-6.9705, -24.7167) projected
  line L230 (-6.9705, -24.7167) -> (-6.6377, -24.6345) projected
  line L231 (-6.6377, -24.6345) -> (-6.2984, -24.5849) projected
  line L232 (-6.2984, -24.5849) -> (-5.956, -24.5683) projected
  line L233 (-5.956, -24.5683) -> (-5.6136, -24.5849) projected
  line L234 (-5.6136, -24.5849) -> (-5.2744, -24.6345) projected
  line L235 (-5.2744, -24.6345) -> (-4.9416, -24.7167) projected
  line L236 (-4.9416, -24.7167) -> (-4.6183, -24.8306) projected
  line L237 (-4.6183, -24.8306) -> (-4.3075, -24.9753) projected
  line L238 (-4.3075, -24.9753) -> (-4.0121, -25.1494) projected
  line L239 (-4.0121, -25.1494) -> (-3.735, -25.3512) projected
  line L240 (-3.735, -25.3512) -> (-3.4787, -25.5788) projected
  line L241 (-3.4787, -25.5788) -> (-3.2455, -25.8302) projected
  line L242 (-3.2455, -25.8302) -> (-3.0378, -26.1029) projected
  line L243 (-3.0378, -26.1029) -> (-2.8574, -26.3944) projected
  line L244 (-2.8574, -26.3944) -> (-2.706, -26.702) projected
  line L245 (-2.706, -26.702) -> (8.32, -26.702) projected
  line L246 (8.32, -26.702) -> (8.4713, -26.3944) projected
  line L247 (8.4713, -26.3944) -> (8.6517, -26.1029) projected
  line L248 (8.6517, -26.1029) -> (8.8595, -25.8302) projected
  line L249 (8.8595, -25.8302) -> (9.0926, -25.5788) projected
  line L250 (9.0926, -25.5788) -> (9.3489, -25.3512) projected
  line L251 (9.3489, -25.3512) -> (9.6261, -25.1494) projected
  line L252 (9.6261, -25.1494) -> (9.9214, -24.9753) projected
  line L253 (9.9214, -24.9753) -> (10.2322, -24.8306) projected
  line L254 (10.2322, -24.8306) -> (10.5555, -24.7167) projected
  line L255 (10.5555, -24.7167) -> (10.8883, -24.6345) projected
  line L256 (10.8883, -24.6345) -> (11.2276, -24.5849) projected
  line L257 (11.2276, -24.5849) -> (11.57, -24.5683) projected
  line L258 (11.57, -24.5683) -> (11.9124, -24.5849) projected
  line L259 (11.9124, -24.5849) -> (12.2516, -24.6345) projected
  line L260 (12.2516, -24.6345) -> (12.5844, -24.7167) projected
  line L261 (12.5844, -24.7167) -> (12.9077, -24.8306) projected
  line L262 (12.9077, -24.8306) -> (13.2185, -24.9753) projected
  line L263 (13.2185, -24.9753) -> (13.5139, -25.1494) projected
  line L264 (13.5139, -25.1494) -> (13.791, -25.3512) projected
  line L265 (13.791, -25.3512) -> (14.0473, -25.5788) projected
  line L266 (14.0473, -25.5788) -> (14.2805, -25.8302) projected
  line L267 (14.2805, -25.8302) -> (14.4882, -26.1029) projected
  line L268 (14.4882, -26.1029) -> (14.6686, -26.3944) projected
  line L269 (14.6686, -26.3944) -> (14.82, -26.702) projected
  line L270 (14.82, -26.702) -> (16.24, -26.702) projected
  line L271 (16.24, -26.702) -> (16.5722, -26.6911) projected
  line L272 (16.5722, -26.6911) -> (16.903, -26.6585) projected
  line L273 (16.903, -26.6585) -> (17.231, -26.6044) projected
  line L274 (17.231, -26.6044) -> (17.5548, -26.5289) projected
  line L275 (17.5548, -26.5289) -> (17.8729, -26.4324) projected
  line L276 (17.8729, -26.4324) -> (18.184, -26.3153) projected
  line L277 (18.184, -26.3153) -> (18.4868, -26.1781) projected
  line L278 (18.4868, -26.1781) -> (18.78, -26.0214) projected
  line L279 (18.78, -26.0214) -> (19.0623, -25.8458) projected
  line L280 (19.0623, -25.8458) -> (19.3325, -25.6522) projected
  line L281 (19.3325, -25.6522) -> (19.5894, -25.4413) projected
  line L282 (19.5894, -25.4413) -> (19.8321, -25.2141) projected
  line L283 (19.8321, -25.2141) -> (20.0593, -24.9715) projected
  line L284 (20.0593, -24.9715) -> (20.2702, -24.7145) projected
  line L285 (20.2702, -24.7145) -> (20.4638, -24.4443) projected
  line L286 (20.4638, -24.4443) -> (20.6394, -24.162) projected
  line L287 (20.6394, -24.162) -> (20.7961, -23.8688) projected
  line L288 (20.7961, -23.8688) -> (20.9333, -23.566) projected
  line L289 (20.9333, -23.566) -> (21.0504, -23.2549) projected
  line L290 (21.0504, -23.2549) -> (21.1469, -22.9368) projected
  line L291 (21.1469, -22.9368) -> (21.2224, -22.613) projected
  line L292 (21.2224, -22.613) -> (21.2765, -22.285) projected
  line L293 (21.2765, -22.285) -> (21.3091, -21.9542) projected
  line L294 (21.3091, -21.9542) -> (21.32, -21.622) projected
  line L295 (21.32, -21.622) -> (21.32, -3.38) projected
  line L296 (21.32, -3.38) -> (20.9643, -3.2049) projected
  line L297 (20.9643, -3.2049) -> (20.6272, -2.9963) projected
  line L298 (20.6272, -2.9963) -> (20.3119, -2.7561) projected
  line L299 (20.3119, -2.7561) -> (20.0212, -2.4866) projected
  line L300 (20.0212, -2.4866) -> (19.758, -2.1902) projected
  line L301 (19.758, -2.1902) -> (19.5247, -1.8697) projected
  line L302 (19.5247, -1.8697) -> (19.3234, -1.5282) projected
  line L303 (19.3234, -1.5282) -> (19.1561, -1.1688) projected
  line L304 (19.1561, -1.1688) -> (19.0243, -0.795) projected
  line L305 (19.0243, -0.795) -> (18.9293, -0.4101) projected
  line L306 (18.9293, -0.4101) -> (18.872, -0.0179) projected
  line L307 (18.872, -0.0179) -> (18.8528, 0.378) projected
  line L308 (18.8528, 0.378) -> (18.872, 0.774) projected
  line L309 (18.872, 0.774) -> (18.9293, 1.1662) projected
  line L310 (18.9293, 1.1662) -> (19.0243, 1.551) projected
  line L311 (19.0243, 1.551) -> (19.1561, 1.9249) projected
  line L312 (19.1561, 1.9249) -> (19.3234, 2.2843) projected
  line L313 (19.3234, 2.2843) -> (19.5247, 2.6258) projected
  line L314 (19.5247, 2.6258) -> (19.758, 2.9462) projected
  line L315 (19.758, 2.9462) -> (20.0212, 3.2426) projected
  line L316 (20.0212, 3.2426) -> (20.3119, 3.5122) projected
  line L317 (20.3119, 3.5122) -> (20.6272, 3.7524) projected
  line L318 (20.6272, 3.7524) -> (20.9643, 3.961) projected
  line L319 (20.9643, 3.961) -> (21.32, 4.136) projected
  line L320 (21.32, 4.136) -> (21.32, 6.0009) projected
  line L321 (21.32, 6.0009) -> (21.2768, 6.303) projected
  line L322 (21.2768, 6.303) -> (21.214, 6.6016) projected
  line L323 (21.214, 6.6016) -> (21.1318, 6.8954) projected
  line L324 (21.1318, 6.8954) -> (21.0306, 7.1833) projected
  line L325 (21.0306, 7.1833) -> (20.9107, 7.4639) projected
  line L326 (20.9107, 7.4639) -> (20.7727, 7.736) projected
  line L327 (20.7727, 7.736) -> (20.6173, 7.9986) projected
  line L328 (20.6173, 7.9986) -> (20.445, 8.2504) projected
  line L329 (20.445, 8.2504) -> (20.2566, 8.4904) projected
  line L330 (20.2566, 8.4904) -> (20.0529, 8.7176) projected
  line L331 (20.0529, 8.7176) -> (19.8348, 8.931) projected
  line L332 (19.8348, 8.931) -> (19.6032, 9.1297) projected
  line L333 (19.6032, 9.1297) -> (19.3591, 9.3127) projected
  line L334 (19.3591, 9.3127) -> (19.1035, 9.4795) projected
  line L335 (19.1035, 9.4795) -> (18.8376, 9.6291) projected
  line L336 (18.8376, 9.6291) -> (18.5625, 9.761) projected
  line L337 (18.5625, 9.761) -> (18.2793, 9.8747) projected
  line L338 (18.2793, 9.8747) -> (17.9893, 9.9696) projected
  line L339 (17.9893, 9.9696) -> (17.6937, 10.0453) projected
  line L340 (17.6937, 10.0453) -> (17.3938, 10.1016) projected
  line L341 (17.3938, 10.1016) -> (17.0909, 10.1381) projected
  line L342 (17.0909, 10.1381) -> (16.7862, 10.1547) projected
  line L343 (16.7862, 10.1547) -> (16.4811, 10.1513) projected
  line L344 (16.4811, 10.1513) -> (16.1769, 10.128) projected
  line L345 (16.1769, 10.128) -> (15.328, 10.128) projected
  line L346 (15.328, 10.128) -> (15.1529, 9.7724) projected
  line L347 (15.1529, 9.7724) -> (14.9443, 9.4353) projected
  line L348 (14.9443, 9.4353) -> (14.7041, 9.1199) projected
  line L349 (14.7041, 9.1199) -> (14.4346, 8.8293) projected
  line L350 (14.4346, 8.8293) -> (14.1382, 8.5661) projected
  line L351 (14.1382, 8.5661) -> (13.8177, 8.3328) projected
  line L352 (13.8177, 8.3328) -> (13.4762, 8.1315) projected
  line L353 (13.4762, 8.1315) -> (13.1168, 7.9642) projected
  line L354 (13.1168, 7.9642) -> (12.743, 7.8324) projected
  line L355 (12.743, 7.8324) -> (12.3581, 7.7374) projected
  line L356 (12.3581, 7.7374) -> (11.9659, 7.68) projected
  line L357 (11.9659, 7.68) -> (11.57, 7.6608) projected
  line L358 (11.57, 7.6608) -> (11.174, 7.68) projected
  line L359 (11.174, 7.68) -> (10.7818, 7.7374) projected
  line L360 (10.7818, 7.7374) -> (10.397, 7.8324) projected
  line L361 (10.397, 7.8324) -> (10.0231, 7.9642) projected
  line L362 (10.0231, 7.9642) -> (9.6637, 8.1315) projected
  line L363 (9.6637, 8.1315) -> (9.3222, 8.3328) projected
  line L364 (9.3222, 8.3328) -> (9.0018, 8.5661) projected
  line L365 (9.0018, 8.5661) -> (8.7054, 8.8293) projected
  line L366 (8.7054, 8.8293) -> (8.4358, 9.1199) projected
  line L367 (8.4358, 9.1199) -> (8.1956, 9.4353) projected
  line L368 (8.1956, 9.4353) -> (7.987, 9.7724) projected
  line L369 (7.987, 9.7724) -> (7.812, 10.128) projected
  line L370 (7.812, 10.128) -> (-10.43, 10.128) projected
  line L371 (-10.43, 10.128) -> (-10.7623, 10.1172) projected
  line L372 (-10.7623, 10.1172) -> (-11.0931, 10.0846) projected
  line L373 (-11.0931, 10.0846) -> (-11.4211, 10.0304) projected
  line L374 (-11.4211, 10.0304) -> (-11.7448, 9.9549) projected
  line L375 (-11.7448, 9.9549) -> (-12.0629, 9.8584) projected
  line L376 (-12.0629, 9.8584) -> (-12.3741, 9.7413) projected
  line L377 (-12.3741, 9.7413) -> (-12.6769, 9.6041) projected
  line L378 (-12.6769, 9.6041) -> (-12.97, 9.4474) projected
  line L379 (-12.97, 9.4474) -> (-13.2523, 9.2719) projected
  line L380 (-13.2523, 9.2719) -> (-13.5225, 9.0783) projected
  line L381 (-13.5225, 9.0783) -> (-13.7795, 8.8674) projected
  circle A0 centre (18.526, 7.08) radius 0.9814
  circle A1 centre (-12.97, -24.162) radius 0.9814
  point P0 (0, 0)
  constraints: 6 tangent, 2 centre point
body "Solid1"
